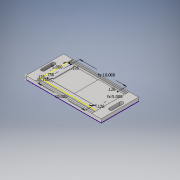
# Autodesk Inventor part: Pedestal Fixture Base
Saved by Autodesk Inventor 2018 (Build 220112000, 112)
## iProperties
Created: 2017-07-11
Part Number: Pedestal Fixture Base
Material: Generic
Document SubType Name: Modeling
Designer: Samuel Clay
Density: 1 g/cm^3
Appearance: Default
Author: Samuel Clay
Autodesk Inventor part; units mm, degrees
ref_plane "YZ Plane" through (0, 0, 0) normal (1, 0, 0) x (0, 1, 0)
ref_plane "XY Plane" through (0, 0, 0) normal (0, 0, 1) x (1, 0, 0)
sketch "Sketch1" plane through (0, 0, 0) normal (0, 1, 0) x (-1, 0, 0)
  line L0 (0, 0) -> (-50.8, 0)
  line L1 (-406.4, 0) -> (-406.4, -203.2)
  line L2 (-406.4, -203.2) -> (-355.6, -203.2)
  line L3 (0, -203.2) -> (0, 0)
  line L4 (-50.8, -203.2) -> (-50.8, 0)
  line L5 (-355.6, -203.2) -> (-355.6, 0)
  line L6 (-50.8, 0) -> (-355.6, 0)
  line L7 (-355.6, 0) -> (-406.4, 0)
  line L8 (-50.8, -203.2) -> (0, -203.2)
  line L9 (-355.6, -203.2) -> (-50.8, -203.2)
  dimension "d0" = 406.4
  dimension "d1" = 203.2
  dimension "d2" = 50.8
  dimension "d3" = 50.8
  constraints: 20 end point, 10 parallel, 9 perpendicular, 3 horizontal, 1 point on line
  measures "d0" distance of L3.start L1.end
  measures "d1" distance of L1.end L1.start
  measures "d2" distance between parallel lines of L4 L3
  measures "d3" distance between parallel lines of L1 L5
sketch "Sketch2" plane through (0, 0, 0) normal (0, 1, 0) x (-1, 0, 0)
  line L0 (-19.05, -139.7) -> (-19.05, -63.5) construction
  line L1 (-9.525, -130.175) -> (-9.525, -73.025)
  line L2 (-28.575, -73.025) -> (-28.575, -130.175)
  arc A0 (-28.575, -130.175) -> (-9.525, -130.175) centre (-19.05, -130.175) ccw
  arc A1 (-9.525, -73.025) -> (-28.575, -73.025) centre (-19.05, -73.025) ccw
  line L3 (-406.4, -203.2) -> (0, -203.2) projected
  line L4 (0, 0) -> (-406.4, 0) projected
  line L5 (0, -203.2) -> (0, 0) projected
  line L6 (-406.4, 0) -> (-406.4, -203.2) projected
  line L7 (-387.35, -139.7) -> (-387.35, -63.5) construction
  line L8 (-377.825, -130.175) -> (-377.825, -73.025)
  line L9 (-396.875, -73.025) -> (-396.875, -130.175)
  arc A2 (-396.875, -130.175) -> (-377.825, -130.175) centre (-387.35, -130.175) ccw
  arc A3 (-377.825, -73.025) -> (-396.875, -73.025) centre (-387.35, -73.025) ccw
  point P0 (-19.05, -177.8)
  point P1 (-19.05, -158.75)
  point P2 (-19.05, -44.45)
  point P3 (-19.05, -25.4)
  point P4 (-387.35, -25.4)
  point P5 (-387.35, -44.45)
  point P6 (-387.35, -158.75)
  point P7 (-387.35, -177.8)
  point P8 (-19.05, -101.6)
  point P9 (-387.35, -101.6)
  dimension "d5" = 19.05
  dimension "d6" = 25.4
  dimension "d7" = 19.05
  dimension "d8" = 19.05
  dimension "d9" = 19.05
  dimension "d10" = 19.05
  dimension "d11" = 19.05
  dimension "d12" = 25.4
  dimension "d13" = 19.05
  dimension "d14" = 76.2
  dimension "d15" = 19.05
  dimension "d16" = 19.05
  dimension "d17" = 19.05
  dimension "d18" = 25.4
  dimension "d19" = 19.05
  dimension "d21" = 19.05
  dimension "d22" = 19.05
  dimension "d25" = 19.05
  dimension "d26" = 19.05
  dimension "d27" = 19.05
  dimension "d28" = 25.4
  dimension "d29" = 19.05
  dimension "d30" = 19.05
  dimension "d31" = 19.05
  dimension "d32" = 76.2
  constraints: 16 end point, 12 point on circle, 8 tangent, 4 centre point, 4 point on line, 2 midpoint, 2 parallel, 1 vertical
  measures "d5" diameter of A1
  measures "d6" distance from line of point (-19.05, -177.8) L3
  measures "d7" distance from line of L5 point (-19.05, -177.8)
  measures "d8" distance of point (-19.05, -177.8) point (-19.05, -158.75)
  measures "d9" distance from line of L5 point (-19.05, -158.75)
  measures "d10" distance from line of L5 point (-19.05, -44.45)
  measures "d11" distance from line of L5 point (-19.05, -25.4)
  measures "d12" distance from line of L4 point (-19.05, -25.4)
  measures "d13" distance of point (-19.05, -25.4) point (-19.05, -44.45)
  measures "d14" distance of L0.start L0.end
  measures "d15" distance of point (-19.05, -158.75) L0.start
  measures "d16" distance of point (-19.05, -44.45) L0.end
  measures "d17" distance from line of L5 point (-19.05, -101.6)
  measures "d18" distance from line of point (-387.35, -177.8) L3
  measures "d19" distance of point (-387.35, -158.75) point (-387.35, -177.8)
  measures "d21" distance from line of L6 point (-387.35, -177.8)
  measures "d22" distance from line of L6 point (-387.35, -158.75)
  measures "d25" distance of point (-387.35, -25.4) point (-387.35, -44.45)
  measures "d26" distance from line of L6 point (-387.35, -44.45)
  measures "d27" distance from line of L6 point (-387.35, -25.4)
  measures "d28" distance from line of L4 point (-387.35, -25.4)
  measures "d29" diameter of A3
  measures "d30" distance of point (-387.35, -158.75) L7.start
  measures "d31" distance of L7.end point (-387.35, -44.45)
  measures "d32" distance of L7.end L7.start
extrude "Extrusion1" add sketch "Sketch1" along normal blind 18.796 contours L3 L8 L4 L0 | L5 L2 L1 L7
extrude "Extrusion2" add sketch "Sketch1" along normal blind 19.05 contours L4 L9 L5 L6
extrude "Extrusion3" cut sketch "Sketch2" along normal through all contours A0 L2 A1 L1 | A2 L9 A3 L8
ref_plane "Work Plane1" through (50.8, 19.05, 0) normal (0, 1, 0) x (-1, 0, 0)
sketch "Pocket Level Sketch" plane through (0, 19.05, 0) normal (0, 1, 0) x (1, 0, 0)
  line L0 (355.6, 203.2) -> (355.6, 0) projected
  line L1 (50.8, 6.35) -> (355.6, 6.35)
  line L2 (355.6, 6.35) -> (355.6, 25.908)
  line L3 (355.6, 25.908) -> (50.8, 25.908)
  line L4 (50.8, 25.908) -> (50.8, 6.35)
  line L5 (50.8, 203.2) -> (50.8, 0) projected
  line L6 (50.8, 196.85) -> (355.6, 196.85)
  line L7 (355.6, 196.85) -> (355.6, 177.292)
  line L8 (355.6, 177.292) -> (50.8, 177.292)
  line L9 (50.8, 177.292) -> (50.8, 196.85)
  line L10 (355.6, 203.2) -> (50.8, 203.2) projected
  line L11 (50.8, 0) -> (355.6, 0) projected
  line L12 (88.9, 44.958) -> (215.9, 44.958)
  line L13 (215.9, 44.958) -> (215.9, 177.292)
  line L14 (215.9, 177.292) -> (88.9, 177.292)
  line L15 (88.9, 177.292) -> (88.9, 44.958)
  circle A0 centre (93.345, 49.403) radius 12.7
  point P0 (0, 0)
  dimension "d39" = 19.558
  dimension "d40" = 6.35
  dimension "d41" = 19.558
  dimension "d42" = 6.35
  dimension "d44" = 38.1
  dimension "d45" = 19.05
  dimension "d46" = 127
  dimension "d50" = 25.4
  dimension "d51" = 4.445
  dimension "d52" = 4.445
  constraints: 24 end point, 6 parallel, 3 horizontal, 3 perpendicular, 3 point on line, 2 collinear, 1 centre point
  measures "d39" distance of L2.end L1.end
  measures "d40" distance between parallel lines of L6 L10
  measures "d41" distance between parallel lines of L6 L8
  measures "d42" distance between parallel lines of L11 L1
  measures "d44" distance between parallel lines of L5 L15
  measures "d45" distance between parallel lines of L3 L12
  measures "d46" distance between parallel lines of L15 L13
  measures "d50" diameter of A0
  measures "d51" distance from line of L12 A0.centre
  measures "d52" distance from line of L15 A0.centre
extrude "Extrusion4" cut sketch "Pocket Level Sketch" against normal blind 3.175 contours L13 L12 A0 L15 L8 | A0 L12 L15 | L15 L12 A0
extrude "Extrusion5" cut sketch "Pocket Level Sketch" against normal blind 10.16 contours L0 L8 L5 L6 | L0 L1 L4 L3
sketch "Origin Sketch" plane through (50.8, 19.05, 0) normal (0, 1, 0) x (-1, 0, 0)
  line L0 (0, -177.292) -> (0, -25.908) projected
  line L1 (0, -25.908) -> (-304.8, -25.908) projected
  circle A0 centre (-19.05, -171.958) radius 1.6002
  circle A1 centre (-273.05, -171.958) radius 1.6002
  circle A2 centre (-273.05, -44.958) radius 1.6002
  circle A3 centre (-19.05, -44.958) radius 1.6002
  point P0 (50.8, 0)
  dimension "d55" = 19.05
  dimension "d56" = 19.05
  dimension "d57" = 3.2004
  dimension "d58" = 3.2004
  dimension "d59" = 3.2004
  dimension "d60" = 127
  dimension "d61" = 127
  dimension "d62" = 254
  dimension "d63" = 254
  dimension "d64" = 3.2004
  constraints: 4 centre point, 1 coincident, 1 horizontal alignment, 1 vertical alignment
  measures "d55" distance from line of L0 point (-19.05, -44.958)
  measures "d56" distance from line of L1 point (-19.05, -44.958)
  measures "d57" diameter of A0
  measures "d58" diameter of A1
  measures "d59" diameter of A2
  measures "d60" distance of point (-19.05, -44.958) A0.centre
  measures "d61" vertical distance of point (-19.05, -44.958) A1.centre
  measures "d62" distance of point (-19.05, -44.958) A2.centre
  measures "d63" horizontal distance of point (-19.05, -44.958) A1.centre
  measures "d64" diameter of A3
extrude "Extrusion6" cut sketch "Origin Sketch" against normal blind 2.54
equation "\"d7\" = d17"
equation "\"d10\" = d7"
equation "\"d11\" = d10"
equation "\"d12\" = d6"
equation "\"d13\" = d8"
equation "\"d15\" = d8"
equation "\"d16\" = d13"
equation "\"d17\" = d9"
equation "\"d18\" = d6"
equation "\"d19\" = d8"
equation "\"d21\" = d9"
equation "\"d22\" = d21"
equation "\"d25\" = d13"
equation "\"d26\" = d22"
equation "\"d27\" = d21"
equation "\"d28\" = d12"
equation "\"d30\" = d19"
equation "\"d31\" = d30"
equation "\"d32\" = d14"
equation "\"d40\" = d42"
equation "\"d41\" = d39"
equation "\"d52\" = d51"
equation "\"d61\" = d60"
equation "\"d63\" = d62"
body "Solid1"
